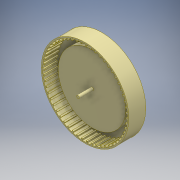
# Autodesk Inventor part: Molde
Saved by Autodesk Inventor 2016 (Build 200138000, 138)
## iProperties
Created: 2019-03-15
Part Number: Molde
Material: Nilón 6/6
Document SubType Name: Modeling
Designer: FIMCP
Density: 1.13 g/cm^3
Appearance: Nilón 6
Mass: 12.4702 g
Surface Area: 104.787 cm^2
Volume: 11.0356 cm^3
Author: FIMCP
Autodesk Inventor part; units mm, degrees
ref_plane "YZ Plane" through (0, 0, 0) normal (1, 0, 0) x (0, 1, 0)
ref_plane "XZ Plane" through (0, 0, 0) normal (0, 1, 0) x (-1, 0, 0)
ref_plane "XY Plane" through (0, 0, 0) normal (0, 0, 1) x (1, 0, 0)
sketch "Boceto1" plane through (0, 0, 0) normal (0, 1, 0) x (-1, 0, 0)
  circle A0 centre (0, 0) radius 31
  circle A1 centre (0, 0) radius 23
  dimension "d0" = 62
  dimension "d35" = 46
  constraints: 2 centre point, 2 coincident
  measures "d0" diameter of A0
  measures "d35" diameter of A1
extrude "Extrusión1" add sketch "Boceto1" along normal blind 2 contours A0 | A1
sketch "Boceto2" plane through (0, 0, 0) normal (0, 1, 0) x (-1, 0, 0)
  circle A0 centre (0, 0) radius 31
  circle A1 centre (0, 0) radius 30
  circle A2 centre (0, 0) radius 1
  dimension "d3" = 62
  dimension "d4" = 60
  dimension "d5" = 2
  constraints: 3 centre point, 3 coincident
  measures "d3" diameter of A0
  measures "d4" diameter of A1
  measures "d5" diameter of A2
extrude "Extrusión2" add sketch "Boceto2" against normal blind 10
sketch "Boceto4" plane through (0, 0, 0) normal (0, 1, 0) x (-1, 0, 0)
  circle A0 centre (0, 0) radius 30 projected
  line L0 (0, 30) -> (-1, 30)
  line L1 (-1, 30) -> (-1, 29)
  line L2 (-1, 29) -> (0, 29)
  line L3 (0, 29) -> (0, 30)
  dimension "d8" = 1
  dimension "d9" = 1
  constraints: 8 end point, 2 parallel, 1 horizontal, 1 perpendicular, 1 vertical alignment, 1 other
  measures "d8" distance of L2.end L1.end
  measures "d9" distance of L1.end L0.end
extrude "Extrusión3" add sketch "Boceto4" against normal blind 10 contours L3 L2 L1 A0 | A0 L1 L0 picked at (-0.5556, 29.3309)
pattern_circular "Patrón circular1" count 55 over 360 about axis through (0, -10, 0) along (0, 1, 0) of "Extrusión3"
sketch "Boceto6" plane through (0, 0, 0) normal (0, 1, 0) x (-1, 0, 0)
  circle A0 centre (0, 0) radius 1 projected
  circle A1 centre (0, 0) radius 1
  dimension "d26" = 2
  constraints: 1 centre point, 1 coincident
  measures "d26" diameter of A1
extrude "Extrusión5" add sketch "Boceto6" against normal blind 15
sketch "Boceto7" plane through (0, 0, 0) normal (0, 1, 0) x (-1, 0, 0)
  circle A0 centre (0, 0) radius 1 projected
  circle A1 centre (0, 0) radius 24
  dimension "d29" = 48
  constraints: 1 centre point, 1 coincident
  measures "d29" diameter of A1
extrude "Extrusión6" add sketch "Boceto7" against normal blind 5
sketch "Boceto8" plane through (0, 0, 0) normal (0, 1, 0) x (-1, 0, 0)
  circle A0 centre (0, 0) radius 1 projected
  circle A1 centre (0, 0) radius 23
  dimension "d32" = 46
  constraints: 1 centre point, 1 coincident
  measures "d32" diameter of A1
extrude "Extrusión7" cut sketch "Boceto8" against normal blind 3
